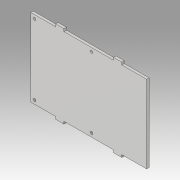
# Autodesk Inventor part: bottom_instrumentboard
Saved by Autodesk Inventor 2019.3 (Build 233278000, 278)
## iProperties
Created: 2019-05-28
Part Number: bottom_instrumentboard
Material: Generic
Document SubType Name: Modeling
Designer: Dave
Density: 1 g/cm^3
Appearance: Default
Author: Dave
Autodesk Inventor part; units mm, degrees
ref_plane "YZ Plane" through (0, 0, 0) normal (1, 0, 0) x (0, 1, 0)
ref_plane "XZ Plane" through (0, 0, 0) normal (0, 1, 0) x (-1, 0, 0)
ref_plane "XY Plane" through (0, 0, 0) normal (0, 0, 1) x (1, 0, 0)
sketch "Sketch1" plane through (0, 0, 0) normal (0, 0, 1) x (1, 0, 0)
  line L0 (0, 0) -> (140, 0)
  line L1 (140, 0) -> (140, 94)
  line L2 (140, 94) -> (0, 94)
  line L3 (0, 94) -> (0, 0)
  circle A0 centre (4.5, 89.5) radius 1.55
  circle A1 centre (4.5, 4.5) radius 1.55
  circle A2 centre (73.5, 89.5) radius 1.55
  circle A3 centre (73.5, 4.5) radius 1.55
  line L4 (0, 69) -> (0, 79)
  line L5 (0, 15) -> (0, 25)
  line L6 (140, 69) -> (140, 79)
  line L7 (140, 15) -> (140, 25)
  line L8 (30, 94) -> (40, 94)
  line L9 (40, 94) -> (40, 97)
  line L10 (40, 97) -> (30, 97)
  line L11 (30, 97) -> (30, 94)
  line L12 (100, 94) -> (110, 94)
  line L13 (110, 94) -> (110, 97)
  line L14 (110, 97) -> (100, 97)
  line L15 (100, 97) -> (100, 94)
  line L16 (30, 0) -> (40, 0)
  line L17 (40, 0) -> (40, -3)
  line L18 (40, -3) -> (30, -3)
  line L19 (30, -3) -> (30, 0)
  line L20 (100, 0) -> (110, 0)
  line L21 (110, 0) -> (110, -3)
  line L22 (110, -3) -> (100, -3)
  line L23 (100, -3) -> (100, 0)
  dimension "d0" = 3.1
  dimension "d1" = 85
  dimension "d2" = 69
  dimension "d3" = 94
  dimension "d4" = 4.5
  dimension "d5" = 4.5
  dimension "d6" = 4.5
  dimension "d7" = 140
  dimension "d12" = 30
  dimension "d13" = 30
  dimension "d16" = 10
  dimension "d17" = 3
  dimension "d18" = 10
  dimension "d19" = 3
  constraints: 48 end point, 13 point on line, 10 parallel, 5 horizontal, 5 perpendicular, 4 centre point, 3 equal radius, 2 collinear, 2 horizontal alignment, 2 vertical alignment
  measures "d0" diameter of A0
  measures "d1" distance of A1.centre A0.centre
  measures "d2" distance of A2.centre A0.centre
  measures "d3" distance between parallel lines of L0 L2
  measures "d4" distance from line of L0 A1.centre
  measures "d5" distance from line of L2 A0.centre
  measures "d6" distance from line of L3 A0.centre
  measures "d7" distance between parallel lines of L1 L3
  measures "d12" distance between parallel lines of L3 L11
  measures "d13" distance between parallel lines of L1 L13
  measures "d16" distance of L9.end L10.end
  measures "d17" distance of L8.end L9.end
  measures "d18" distance of L17.end L18.end
  measures "d19" distance of L16.end L17.end
extrude "Extrusion1" add sketch "Sketch1" along normal blind 3
body "Solid1"
